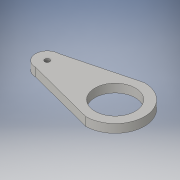
# Autodesk Inventor part: Light_Hooker
Saved by Autodesk Inventor 2016 (Build 200138000, 138)
## iProperties
Created: 2019-03-08
Part Number: Light_Hooker
Material: Generic
Document SubType Name: Modeling
Designer: student
Density: 1 g/cm^3
Appearance: Default
Author: student
Autodesk Inventor part; units mm, degrees
ref_plane "YZ Plane" through (0, 0, 0) normal (1, 0, 0) x (0, 1, 0)
ref_plane "XZ Plane" through (0, 0, 0) normal (0, 1, 0) x (-1, 0, 0)
ref_plane "XY Plane" through (0, 0, 0) normal (0, 0, 1) x (1, 0, 0)
sketch "Sketch1" plane through (0, 0, 0) normal (0, 1, 0) x (-1, 0, 0)
  circle A0 centre (0, 0) radius 10.922
  arc A1 (0, 15.875) -> (0, -15.875) centre (0, 0) ccw
  line L0 (0, 0) -> (36.703, 0) construction
  arc A2 (36.703, -6.35) -> (36.703, 6.35) centre (36.703, 0) ccw
  line L1 (0, 15.875) -> (36.703, 6.35)
  line L2 (0, -15.875) -> (36.703, -6.35)
  circle A3 centre (36.703, 0) radius 1.3335
  dimension "d0" = 21.844
  dimension "d1" = 31.75
  dimension "d2" = 36.703
  dimension "d3" = 12.7
  dimension "d4" = 2.667
  constraints: 6 end point, 4 centre point, 4 coincident, 4 point on circle, 1 horizontal
  measures "d0" diameter of A0
  measures "d1" diameter of A1
  measures "d2" distance of L0.start L0.end
  measures "d3" diameter of A2
  measures "d4" diameter of A3
extrude "Extrusion1" add sketch "Sketch1" along normal blind 4.572
body "Solid1"
